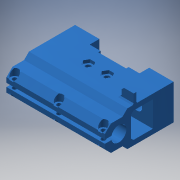
# Autodesk Inventor part: XEndBushingLeft
Saved by Autodesk Inventor 2016 (Build 200138000, 138)
## iProperties
Category: Print
Created: 2014-08-15
Part Number: XEndBushingLeft
Material: ABS Plastic
Document SubType Name: Modeling
Designer: t_clevj
Density: 1.06 g/cm^3
Appearance: Cyan
Mass: 65.1875 g
Surface Area: 259.038 cm^2
Volume: 61.4976 cm^3
Vendor: Jack
Author: Jack
Title: X End Left
Autodesk Inventor part; units mm, degrees
ref_plane "YZ Plane" through (0, 0, 0) normal (1, 0, 0) x (0, 1, 0)
ref_plane "XZ Plane" through (0, 0, 0) normal (0, 1, 0) x (-1, 0, 0)
ref_plane "XY Plane" through (0, 0, 0) normal (0, 0, 1) x (1, 0, 0)
sketch "Sketch1" plane through (0, 0, 0) normal (1, 0, 0) x (0, 1, 0)
  arc A0 (-6.0673, -1.5) -> (-6.0673, 1.5) centre (0, 0) ccw
  line L0 (-11.5, 1.5) -> (-11.5, 12.5)
  line L1 (-11.5, 12.5) -> (35, 12.5)
  line L2 (-11.5, -1.5) -> (-11.5, -12.5)
  line L3 (-11.5, -12.5) -> (35, -12.5)
  line L4 (-11.5, 1.5) -> (-6.0673, 1.5)
  line L5 (-11.5, -1.5) -> (-6.0673, -1.5)
  line L6 (35, 12.5) -> (35, -12.5)
  dimension "d0" = 12.5
  dimension "d1" = 1.5
  dimension "d2" = 1.5
  dimension "d3" = 11.5
  dimension "d4" = 12.5
  dimension "d5" = 12.5
  dimension "d140" = 35
  constraints: 14 end point, 3 vertical, 2 horizontal, 2 point on circle, 2 vertical alignment, 1 centre point, 1 coincident, 1 parallel, 1 perpendicular
  measures "d0" diameter of A0
  measures "d1" vertical distance of point (0, 0) L2.start
  measures "d2" vertical distance of point (0, 0) L0.start
  measures "d3" distance from line of point (0, 0) L0
  measures "d4" distance from line of point (0, 0) L1
  measures "d5" distance from line of L3 point (0, 0)
  measures "d140" distance from line of L6 point (0, 0)
extrude "MainBlock" add sketch "Sketch1" along normal blind 81
chamfer "BearingHolderChamfer" distance 5 angle 45 2 edges at (40.5, -11.5, 12.5) (40.5, -11.5, -12.5)
sketch "Sketch2" plane through (0, 35, 12.5) normal (0, 0, 1) x (1, 0, 0)
  line L0 (81, -46.5) -> (81, -41.5) projected
  line L1 (81, -41.5) -> (0, -41.5) projected
  line L2 (0, -41.5) -> (0, -46.5) projected
  line L3 (0, -46.5) -> (81, -46.5) projected
  line L4 (0, -41.5) -> (0, 0) projected
  point P0 (0, -35)
  point P1 (4, -43.75)
  point P2 (77, -43.75)
  point P3 (40.5, -43.75)
  dimension "d17" = 2.75
  dimension "d18" = 4
  dimension "d19" = 4
  dimension "d220" = 40.5
  constraints: 2 horizontal alignment
  measures "d17" distance from line of L3 point (77, -43.75)
  measures "d18" distance from line of L0 point (77, -43.75)
  measures "d19" distance from line of L2 point (4, -43.75)
  measures "d220" distance from line of L4 point (40.5, -43.75)
hole "BearingHolderClamp" at (4, -8.75, 12.5) at (77, -8.75, 12.5) at (40.5, -8.75, 12.5) direction (0, 0, -1) diameter 3.5 depth 25 tip angle 118 counterbore diameter 6.5 counterbore depth 7.75
sketch "Sketch3" plane through (81, 35, -12.5) normal (0, 0, -1) x (-1, 0, 0)
  circle A0 centre (77, -43.75) radius 1.75 projected
  circle A1 centre (77, -43.75) radius 1.75 projected
  circle A2 centre (4, -43.75) radius 1.75 projected
  circle A3 centre (4, -43.75) radius 1.75 projected
  line L0 (7.3486, -43.75) -> (5.6743, -46.65)
  line L1 (5.6743, -46.65) -> (2.3257, -46.65)
  line L2 (2.3257, -46.65) -> (0.6514, -43.75)
  line L3 (0.6514, -43.75) -> (2.3257, -40.85)
  line L4 (2.3257, -40.85) -> (5.6743, -40.85)
  line L5 (5.6743, -40.85) -> (7.3486, -43.75)
  line L6 (80.3486, -43.75) -> (78.6743, -46.65)
  line L7 (78.6743, -46.65) -> (75.3257, -46.65)
  line L8 (75.3257, -46.65) -> (73.6514, -43.75)
  line L9 (73.6514, -43.75) -> (75.3257, -40.85)
  line L10 (75.3257, -40.85) -> (78.6743, -40.85)
  line L11 (78.6743, -40.85) -> (80.3486, -43.75)
  circle A4 centre (40.5, -43.75) radius 1.75 projected
  line L12 (43.8486, -43.75) -> (42.1743, -46.65)
  line L13 (42.1743, -46.65) -> (38.8257, -46.65)
  line L14 (38.8257, -46.65) -> (37.1514, -43.75)
  line L15 (37.1514, -43.75) -> (38.8257, -40.85)
  line L16 (38.8257, -40.85) -> (42.1743, -40.85)
  line L17 (42.1743, -40.85) -> (43.8486, -43.75)
  point P0 (81, -35)
  dimension "d27" = 5.8
  dimension "d28" = 5.8
  constraints: 36 end point, 3 coincident, 3 horizontal, 1 collinear, 39 other
  measures "d27" distance between parallel lines of L1 L4
  measures "d28" distance between parallel lines of L7 L10
extrude "BearingHolderNutTrap" cut sketch "Sketch3" against normal blind 7.75
sketch "Sketch4" plane through (0, 0, 0) normal (-1, 0, 0) x (0, 0, 1)
  arc A0 (1.5, -6.0673) -> (-1.5, -6.0673) centre (0, 0) ccw projected
  line L0 (-12.5, 35) -> (-12.5, -6.5) projected
  line L1 (10.5, 10) -> (-10.5, 10)
  line L2 (-10.5, 10) -> (-10.5, 28)
  line L3 (-10.5, 28) -> (10.5, 28)
  line L4 (10.5, 28) -> (10.5, 10)
  dimension "d31" = 18
  dimension "d32" = 21
  dimension "d33" = 10
  dimension "d34" = 2
  constraints: 8 end point, 2 parallel, 1 horizontal, 1 perpendicular
  measures "d31" distance of L1.end L2.end
  measures "d32" distance of L1.start L1.end
  measures "d33" distance from line of A0.centre L1
  measures "d34" distance between parallel lines of L0 L2
extrude "BeltCutoutY" cut sketch "Sketch4" against normal up to surface (81 mm away)
sketch "Sketch5" plane through (0, 35, 12.5) normal (0, 1, 0) x (1, 0, 0)
  line L0 (81, 25) -> (81, 0) projected
  line L1 (0, 25) -> (81, 25) projected
  line L2 (29, 2) -> (52, 2)
  line L3 (52, 2) -> (52, 23)
  line L4 (52, 23) -> (29, 23)
  line L5 (29, 23) -> (29, 2)
  point P0 (0, 12.5)
  dimension "d37" = 21
  dimension "d38" = 23
  dimension "d39" = 2
  dimension "d40" = 29
  constraints: 8 end point, 2 parallel, 1 horizontal, 1 perpendicular
  measures "d37" distance of L4.end L2.start
  measures "d38" distance of L2.start L2.end
  measures "d39" distance between parallel lines of L1 L4
  measures "d40" distance between parallel lines of L0 L3
extrude "BeltCutoutX" cut sketch "Sketch5" against normal up to surface (7 mm away)
sketch "Sketch6" plane through (81, 35, -12.5) normal (0, 0, -1) x (-1, 0, 0)
  line L0 (81, 0) -> (81, -41.5) projected
  line L1 (81, 0) -> (0, 0) projected
  line L2 (0, -41.5) -> (0, 0) projected
  line L3 (0, -28) -> (81, -28)
  point P0 (81, -35)
  dimension "d43" = 28
  constraints: 2 end point, 2 point on line, 1 perpendicular
  measures "d43" distance between parallel lines of L1 L3
extrude "BoltPadUpper" add sketch "Sketch6" along normal blind 2
sketch "Sketch7" plane through (0, 35, 12.5) normal (0, 0, 1) x (1, 0, 0)
  line L0 (81, 0) -> (81, -41.5) projected
  line L1 (0, 0) -> (81, 0) projected
  line L2 (0, -41.5) -> (0, 0) projected
  line L3 (0, -28) -> (0, 0) projected
  line L4 (0, -28) -> (81, -28)
  line L5 (81, 0) -> (81, -28) projected
  point P0 (0, -35)
  dimension "d46" = 28
  constraints: 2 end point, 2 point on line, 1 perpendicular
  measures "d46" distance between parallel lines of L1 L4
extrude "BoltPadLower" add sketch "Sketch7" along normal blind 2
chamfer "BoltPadChamfer" distance 2 angle 45 2 edges at (40.5, 7, 12.5) (40.5, 7, -12.5)
sketch "Sketch8" plane through (81, 35, -14.5) normal (0, 0, -1) x (-1, 0, 0)
  line L0 (81, 0) -> (0, 0) projected
  line L1 (0, 0) -> (0, -28) projected
  point P0 (81, -35)
  point P1 (32.75, -12)
  point P2 (48.25, -12)
  dimension "d54" = 12
  dimension "d116" = 15.5
  dimension "d117" = 32.75
  constraints: 1 horizontal alignment
  measures "d54" distance from line of L0 point (48.25, -12)
  measures "d116" distance of point (48.25, -12) point (32.75, -12)
  measures "d117" distance from line of L1 point (32.75, -12)
hole "BearingBoltHoles" at (48.25, 23, -14.5) at (32.75, 23, -14.5) direction (0, 0, 1) diameter 4.5 end up to face face through (27, 16.3333, 14.5) facing (0, 0, 1) counterbore diameter 8 counterbore depth 1.5
chamfer "BearingCutoutYChamfer" distance 2 angle 45 2 edges at (40.5, 10, 10.5) (40.5, 10, -10.5)
sketch "Sketch9" plane through (52, 35, 10.5) normal (0, 0, -1) x (-1, 0, 0)
  line L0 (52, -7) -> (23, -7) projected
  line L1 (23, 0) -> (23, -7) projected
  line L2 (0, 0) -> (0, -7) projected
  line L3 (0, -7) -> (-29, -7) projected
  circle A0 centre (19.25, -12) radius 2.25 projected
  circle A1 centre (3.75, -12) radius 2.25 projected
  arc A2 (0, -1.6589) -> (-6.048, -7) centre (3.75, -12) ccw
  arc A3 (29.048, -7) -> (23, -1.6589) centre (19.25, -12) ccw
  line L4 (0, -1.6589) -> (0, -7)
  line L5 (0, -7) -> (-6.048, -7)
  line L6 (23, -1.6589) -> (23, -7)
  line L7 (23, -7) -> (29.048, -7)
  point P0 (52, -35)
  dimension "d67" = 11
  dimension "d68" = 11
  constraints: 8 end point, 4 collinear, 4 point on circle, 4 point on line, 2 centre point, 2 coincident
  measures "d67" radius of A3
  measures "d68" radius of A2
sketch "Sketch10" plane through (0, 35, 14.5) normal (0, 0, 1) x (1, 0, 0)
  circle A0 centre (48.25, -12) radius 2.25 projected
  circle A1 centre (32.75, -12) radius 2.25 projected
  line L0 (37.0224, -12) -> (34.8862, -15.7)
  line L1 (34.8862, -15.7) -> (30.6138, -15.7)
  line L2 (30.6138, -15.7) -> (28.4776, -12)
  line L3 (28.4776, -12) -> (30.6138, -8.3)
  line L4 (30.6138, -8.3) -> (34.8862, -8.3)
  line L5 (34.8862, -8.3) -> (37.0224, -12)
  line L6 (52.5224, -12) -> (50.3862, -15.7)
  line L7 (50.3862, -15.7) -> (46.1138, -15.7)
  line L8 (46.1138, -15.7) -> (43.9776, -12)
  line L9 (43.9776, -12) -> (46.1138, -8.3)
  line L10 (46.1138, -8.3) -> (50.3862, -8.3)
  line L11 (50.3862, -8.3) -> (52.5224, -12)
  point P0 (0, -35)
  dimension "d71" = 7.4
  constraints: 24 end point, 2 coincident, 2 horizontal, 1 collinear, 26 other
  measures "d71" distance between parallel lines of L1 L4
extrude "BearingNutTrap" cut sketch "Sketch10" against normal blind 2.5
sketch "Sketch11" plane through (81, 35, -14.5) normal (0, 0, -1) x (-1, 0, 0)
  line L0 (81, 0) -> (0, 0) projected
  line L1 (0, 10) -> (26, 10)
  line L2 (81, 10) -> (55, 10)
  line L3 (81, 10) -> (81, 0)
  line L4 (0, 0) -> (0, 10)
  line L5 (29, 0) -> (29, 0)
  line L6 (52, 0) -> (52, 0)
  line L7 (29, 0) -> (29, 8)
  line L8 (29, 0) -> (29, -7) projected
  line L9 (52, 0) -> (52, 8)
  line L10 (55, 10) -> (52, 8)
  line L11 (26, 10) -> (29, 8)
  point P0 (81, -35)
  dimension "d74" = 26
  dimension "d75" = 26
  dimension "d80" = 10
  dimension "d93" = 8
  constraints: 20 end point, 2 horizontal, 2 perpendicular, 2 vertical, 1 collinear, 1 horizontal alignment, 1 parallel, 1 point on line
  measures "d74" distance of L1.start L1.end
  measures "d75" distance of L2.start L2.end
  measures "d80" distance of L2.start L0.start
  measures "d93" distance of L5.end L7.end
extrude "XRodHolderPad" add sketch "Sketch11" against normal up to surface (29 mm away)
sketch "Sketch15" plane through (0, 45, -14.5) normal (0, 1, 0) x (1, 0, 0)
  line L0 (55, -29) -> (81, -29) projected
  line L1 (81, 0) -> (81, -29) projected
  line L2 (55, 0) -> (81, 0) projected
  line L3 (55, 0) -> (55, -29) projected
  circle A0 centre (13, -14.5) radius 4.15
  circle A1 centre (68, -14.5) radius 4.15
  line L4 (0, 0) -> (0, -29) projected
  point P0 (0, -14.5)
  dimension "d94" = 8.3
  dimension "d95" = 8.3
  dimension "d99" = 14.5
  dimension "d137" = 13
  dimension "d183" = 13
  constraints: 2 centre point, 1 horizontal alignment
  measures "d94" diameter of A0
  measures "d95" diameter of A1
  measures "d99" distance from line of L0 A1.centre
  measures "d137" distance from line of L1 A1.centre
  measures "d183" distance from line of L4 A0.centre
extrude "XRodHole" cut sketch "Sketch15" against normal up to surface (17 mm away) contours A0 | A1
sketch "Sketch20" plane through (81, 35, -14.5) normal (0, 0, -1) x (-1, 0, 0)
  line L0 (26, 10) -> (0, 10) projected
  line L1 (0, 10) -> (0, -28) projected
  line L2 (81, -28) -> (81, 10) projected
  point P0 (81, -35)
  point P1 (68, 2)
  point P2 (13, 2)
  dimension "d122" = 8
  dimension "d123" = 13
  dimension "d124" = 13
  constraints: 1 horizontal alignment
  measures "d122" distance from line of L0 point (13, 2)
  measures "d123" distance from line of L1 point (13, 2)
  measures "d124" distance from line of L2 point (68, 2)
hole "Hole3" at (13, 37, -14.5) at (68, 37, -14.5) direction (0, 0, 1) diameter 3 depth 10 counterbore diameter 6.5 counterbore depth 3.7
ref_plane "Work Plane3" through (0, 35, -1) normal (0, 0, 1) x (1, 0, 0)
sketch "Sketch21" plane through (0, 35, -1) normal (0, 0, 1) x (1, 0, 0)
  circle A0 centre (13, 2) radius 1.5 projected
  circle A1 centre (68, 2) radius 1.5 projected
  line L0 (13, 5.3486) -> (15.9, 3.6743)
  line L1 (15.9, 3.6743) -> (15.9, 0.3257)
  line L2 (15.9, 0.3257) -> (13, -1.3486)
  line L3 (13, -1.3486) -> (10.1, 0.3257)
  line L4 (10.1, 0.3257) -> (10.1, 3.6743)
  line L5 (10.1, 3.6743) -> (13, 5.3486)
  line L6 (68, 5.3486) -> (70.9, 3.6743)
  line L7 (70.9, 3.6743) -> (70.9, 0.3257)
  line L8 (70.9, 0.3257) -> (68, -1.3486)
  line L9 (68, -1.3486) -> (65.1, 0.3257)
  line L10 (65.1, 0.3257) -> (65.1, 3.6743)
  line L11 (65.1, 3.6743) -> (68, 5.3486)
  point P0 (0, -35)
  dimension "d133" = 5.8
  constraints: 24 end point, 2 coincident, 2 vertical, 1 parallel, 26 other
  measures "d133" distance between parallel lines of L7 L10
extrude "Extrusion18" cut sketch "Sketch21" against normal blind 6 contours A0 | A1 | L0 L1 L2 L3 L4 L5 | L6 L7 L8 L9 L10 L11
extrude "Extrusion19" cut sketch "Sketch9" along normal up to surface (21 mm away) contours L0 L1 A3 | L2 L3 A2
sketch "Sketch27" plane through (29, 35, -10.5) normal (0, 0, 1) x (1, 0, 0)
  circle A0 centre (3.75, -12) radius 2.25 projected
  circle A1 centre (3.75, -12) radius 4.75
  point P0 (-29, -35)
  dimension "d154" = 9.5
  constraints: 1 centre point, 1 coincident
  measures "d154" diameter of A1
extrude "Extrusion25" cut sketch "Sketch27" against normal blind 0.25
sketch "Sketch31" plane through (0, 0, 0) normal (-1, 0, 0) x (0, 0, 1)
  line L0 (-7.5, -11.5) -> (-12.5, -6.5) projected
  arc A0 (1.5, -6.0673) -> (-1.5, -6.0673) centre (0, 0) ccw projected
  line L1 (12.5, -6.5) -> (7.5, -11.5) projected
  line L2 (12.5, -6.5) -> (12.5, 5) projected
  line L3 (14.5, 7) -> (12.5, 5) projected
  line L4 (-12.5, 5) -> (-14.5, 7) projected
  line L5 (-12.5, 5) -> (-12.5, -6.5) projected
  line L6 (-10.5, -8.5) -> (-10.5, 3)
  line L7 (-10.5, 3) -> (-12.5, 5)
  line L8 (10.5, -8.5) -> (10.5, 3)
  line L9 (10.5, 3) -> (12.5, 5)
  dimension "d192" = 10.5
  dimension "d193" = 10.5
  constraints: 8 end point, 2 collinear, 2 point on line, 2 vertical
  measures "d192" distance from line of L6 A0.centre
  measures "d193" distance from line of L8 A0.centre
extrude "Extrusion29" cut sketch "Sketch31" against normal up to next
sketch "Sketch32" plane through (0, 0, 0) normal (-1, 0, 0) x (0, 0, 1)
  line L0 (-7.5, -11.5) -> (-10.5, -8.5) projected
  line L1 (1.5, -11.5) -> (7.5, -11.5) projected
  line L2 (10.5, -8.5) -> (7.5, -11.5) projected
  line L3 (5.5, -11.5) -> (10.5, -6.5)
  line L4 (10.5, -8.5) -> (10.5, -5.5) projected
  line L5 (-1.5, -11.5) -> (-7.5, -11.5) projected
  line L6 (-5.5, -11.5) -> (-10.5, -6.5)
  line L7 (-10.5, -8.5) -> (-10.5, 3) projected
  dimension "d188" = 5
  dimension "d189" = 5
  constraints: 4 end point, 4 point on line, 1 horizontal alignment, 1 perpendicular
  measures "d188" horizontal distance of L3.start L3.end
  measures "d189" horizontal distance of L3.end L3.start
extrude "Extrusion30" cut sketch "Sketch32" against normal up to surface (81 mm away)
sketch "Sketch33" plane through (81, 0, 0) normal (1, 0, 0) x (0, 0, -1)
  line L0 (14.5, 45) -> (-14.5, 45) projected
  line L1 (-14.5, 7) -> (-14.5, 45) projected
  line L2 (-14.5, 14.25) -> (-22.5, 14.25)
  line L3 (-22.5, 14.25) -> (-22.5, 12.25)
  line L4 (-22.5, 12.25) -> (-14.5, 12.25)
  dimension "d194" = 2
  dimension "d195" = 30.75
  dimension "d196" = 8
  constraints: 6 end point, 2 perpendicular, 2 point on line, 1 horizontal
  measures "d194" distance of L2.end L3.end
  measures "d195" distance between parallel lines of L0 L2
  measures "d196" distance of L3.end L4.end
extrude "Extrusion31" add sketch "Sketch33" against normal blind 10
chamfer "Chamfer6" distance 2 angle 45 1 edges at (71, 13.25, 22.5)
chamfer "Chamfer7" distance 5 angle 45 2 edges at (52, 39, -14.5) (29, 39, -14.5)
sketch "Sketch34" plane through (81, 35, -14.5) normal (0, 0, -1) x (-1, 0, 0)
  line L0 (57, 0) -> (57, 10) projected
  line L1 (24, 0) -> (57, 0) projected
  line L2 (53, 0) -> (28, 0) projected
  line L3 (33.5, 0) -> (33.5, -3)
  line L4 (33.5, -3) -> (47.5, -3)
  line L5 (47.5, -3) -> (47.5, 0)
  line L6 (47.5, 0) -> (33.5, 0)
  point P0 (81, -35)
  point P1 (52, 0)
  point P2 (29, 0)
  dimension "d205" = 3
  dimension "d206" = 14
  dimension "d207" = 9.5
  constraints: 8 end point, 3 perpendicular, 2 point on line, 1 collinear
  measures "d205" distance of L4.end L5.end
  measures "d206" distance of L3.end L4.end
  measures "d207" distance between parallel lines of L0 L5
extrude "Extrusion32" cut sketch "Sketch34" against normal up to surface (4 mm away)
sketch "Sketch35" plane through (81, 35, -14.5) normal (0, 0, -1) x (-1, 0, 0)
  line L0 (47.5, -3) -> (33.5, -3) projected
  line L1 (33.5, -3) -> (33.5, 0) projected
  line L2 (39.5, -3) -> (39.5, 5)
  line L3 (39.5, 5) -> (41.5, 5)
  line L4 (41.5, 5) -> (41.5, -3)
  point P0 (81, -35)
  dimension "d210" = 2
  dimension "d211" = 6
  dimension "d212" = 8
  constraints: 6 end point, 2 perpendicular, 2 point on line, 1 vertical
  measures "d210" distance of L2.end L3.end
  measures "d211" distance between parallel lines of L1 L2
  measures "d212" distance of L3.end L4.end
extrude "Extrusion33" add sketch "Sketch35" along normal blind 3 and the other way blind 4
chamfer "Chamfer8" distance 3 angle 45 1 edges at (40.5, 32, -14.5)
chamfer "Chamfer9" distance 1 angle 45 2 edges at (41.5, 32, -12.5) (39.5, 32, -12.5)
chamfer "Chamfer10" distance 2 angle 45 1 edges at (71, 13.25, 14.5)
chamfer "Chamfer11" distance 1 angle 45 4 edges at (70, 12.25, 14.5) (76, 12.25, 14.5) (70, 14.25, 14.5) (76, 14.25, 14.5)
chamfer "Chamfer12" distance 3 angle 45 1 edges at (56, 45, -13.5)
sketch "Sketch36" plane through (0, 45, 14.5) normal (0, 1, 0) x (1, 0, 0)
  line L0 (0, 0) -> (26, 0) projected
  line L1 (29, 24) -> (29, 0) projected
  line L2 (52, 22.5858) -> (52, 0) projected
  line L3 (55, 22.7574) -> (55, 0) projected
  line L4 (29, 0) -> (20, 0)
  line L5 (0, 0) -> (81, 0) projected
  line L6 (20, 0) -> (20, 14.3)
  line L7 (20, 14.3) -> (29, 14.3)
  line L8 (52, 14.3) -> (61, 14.3)
  line L9 (61, 14.3) -> (61, 0)
  line L10 (55, 0) -> (81, 0) projected
  point P0 (0, 14.5)
  dimension "d233" = 9
  dimension "d234" = 14.3
  dimension "d235" = 9
  constraints: 10 end point, 6 point on line, 3 perpendicular
  measures "d233" distance of L1.end L4.end
  measures "d234" distance of L4.end L6.end
  measures "d235" distance of L8.start L8.end
extrude "Extrusion34" cut sketch "Sketch36" against normal blind 8
body "Solid1"
